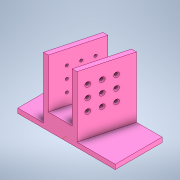
# Autodesk Inventor part: pvcBracketUpperPortion
Saved by Autodesk Inventor 2022.2 (Build 262287000, 287)
## iProperties
Created: 2021-10-20
Part Number: pvcBracketUpperPortion
Material: PC/ABS Plastic
Document SubType Name: Modeling
Designer: robst
Density: 0.357273 g/cm^3
Appearance: Pink
Author: robst
Autodesk Inventor part; units mm, degrees
ref_plane "YZ Plane" through (0, 0, 0) normal (1, 0, 0) x (0, 1, 0)
ref_plane "XZ Plane" through (0, 0, 0) normal (0, 1, 0) x (-1, 0, 0)
ref_plane "XY Plane" through (0, 0, 0) normal (0, 0, 1) x (1, 0, 0)
sketch "Sketch8" plane through (0, 0, 0) normal (0, 1, 0) x (-1, 0, 0)
  line L0 (83, 40) -> (-83, 40)
  line L1 (-83, 40) -> (-83, -40)
  line L2 (-83, -40) -> (83, -40)
  line L3 (83, -40) -> (83, 40)
  line L4 (83, 40) -> (-83, -40) construction
  line L5 (-83, 40) -> (83, -40) construction
  point P0 (0, 0)
  dimension "d28" = 80
  dimension "d29" = 166
  constraints: 12 end point, 2 midpoint, 2 parallel, 1 horizontal, 1 perpendicular
  measures "d28" distance of L2.end L0.start
  measures "d29" distance between parallel lines of L1 L3
extrude "Extrusion8" add sketch "Sketch8" against normal blind 8
sketch "Sketch11" plane through (0, 0, 0) normal (0, 1, 0) x (1, 0, 0)
  line L0 (83, 40) -> (-83, 40) projected
  line L1 (-83, -40) -> (83, -40) projected
  line L2 (-83, 40) -> (-83, -40) projected
  line L3 (83, -40) -> (83, 40) projected
  line L4 (-31.038, -40) -> (-9.602, 40)
  line L5 (-9.602, 40) -> (-17.8842, 40)
  line L6 (-75, 40) -> (75, 40) projected
  line L7 (-17.8842, 40) -> (-39.3202, -40)
  line L8 (-39.3202, -40) -> (-31.038, -40)
  line L9 (-31.038, -40) -> (-31.038, 40) construction
  line L10 (0, -40) -> (0, 40) construction
  line L11 (9.602, -40) -> (31.038, 40)
  line L12 (31.038, 40) -> (39.3202, 40)
  line L13 (39.3202, 40) -> (17.8842, -40)
  line L14 (17.8842, -40) -> (9.602, -40)
  point P0 (0, 0)
  point P1 (0, -40)
  point P2 (0, -40)
  point P3 (-20.32, 0)
  point P4 (0, 0)
  point P5 (20.32, 0)
  point P6 (39.3202, 40)
  point P7 (31.038, 40)
  point P8 (-17.8842, 40)
  dimension "d39" = -15
  dimension "d40" = 8
  dimension "d42" = 8
  dimension "d44" = 20.32
  dimension "d45" = 20.32
  constraints: 20 end point, 5 point on line, 4 midpoint, 3 parallel, 2 horizontal, 1 perpendicular, 8 other
  measures "d39" angle of L4 L9
  measures "d40" distance between parallel lines of L7 L4
  measures "d42" distance between parallel lines of L13 L11
  measures "d44" distance of point (-20.32, 0) point (0, 0)
  measures "d45" distance of point (20.32, 0) point (0, 0)
extrude "Extrusion11" add sketch "Sketch11" along normal blind 104.1375 contours L13 L1 L11 L0 | L4 L1 L7 L0
sketch "Sketch12" plane through (0, 0, 0) normal (0, 1, 0) x (1, 0, 0)
  line L0 (31.038, 40) -> (-9.602, 40) projected
  line L1 (31.038, 40) -> (9.602, -40) projected
  line L2 (-31.038, -40) -> (9.602, -40) projected
  line L3 (-31.038, -40) -> (-9.602, 40) projected
  line L4 (-9.602, 40) -> (31.038, 40)
  line L5 (31.038, 40) -> (9.602, -40)
  line L6 (9.602, -40) -> (-31.038, -40)
  line L7 (-9.602, 40) -> (-31.038, -40) projected
  line L8 (-31.038, -40) -> (-9.602, 40)
  point P0 (0, 0)
  constraints: 8 end point, 3 equal length
extrude "Extrusion12" add sketch "Sketch12" along normal blind 20
sketch "Sketch15" plane through (-39.3202, 0, 40) normal (-0.9659258, 0, -0.258819) x (-0.258819, 0, 0.9659258)
  line L0 (-82.8221, 104.1375) -> (0, 104.1375) projected
  line L1 (0, 0) -> (0, 104.1375) projected
  line L2 (-82.8221, 0) -> (-82.8221, 104.1375) projected
  line L3 (-2.1436, 20) -> (-84.9657, 20) projected
  line L4 (-82.8221, 40) -> (0, 40) construction
  line L5 (-67.8221, 40) -> (-67.8221, 104.1375) construction
  point P0 (-48.8138, 0)
  point P1 (-82.8221, 52.0688)
  point P2 (-47.8221, 40)
  point P3 (-27.8221, 40)
  point P4 (-67.8221, 60)
  point P5 (-47.8221, 60)
  point P6 (-27.8221, 60)
  point P7 (-67.8221, 80)
  point P8 (-47.8221, 80)
  point P9 (-27.8221, 80)
  dimension "d64" = 15
  dimension "d74" = 20
  dimension "d77" = 20
  dimension "d90" = 20
  constraints: 4 end point, 4 point on line, 2 perpendicular, 1 coincident, 1 horizontal, 1 midpoint, 1 vertical, 8 other
  measures "d64" distance from line of point (-82.822, 52.069) L5
  measures "d74" distance of point (-67.822, 40) point (-47.822, 40)
  measures "d77" distance of point (-67.822, 40) point (-67.822, 60)
  measures "d90" distance between parallel lines of L4 L3
hole "HoleForLeftSideOf2x4" at (-21.7665, 40, -25.5111) at (-26.9429, 40, -6.1926) at (-32.1193, 40, 13.1259) at (-26.9429, 60, -6.1926) at (-21.7665, 60, -25.5111) at (-32.1193, 60, 13.1259) at (-32.1193, 80, 13.1259) at (-26.9429, 80, -6.1926) at (-21.7665, 80, -25.5111) direction (0.9659258, 0, 0.258819) diameter 4.496 depth 8 countersink diameter 8.433 countersink angle 82 clearance for "Flat Head Machine Screw (82)" size "#8" standard "Ansi Unified Screw Threads"
sketch "Sketch16" plane through (39.3202, 0, -40) normal (0.9659258, 0, 0.258819) x (0.258819, 0, -0.9659258)
  line L0 (-82.8221, 104.1375) -> (0, 104.1375) projected
  line L1 (0, 0) -> (0, 104.1375) projected
  line L2 (-82.8221, 0) -> (-82.8221, 104.1375) projected
  line L3 (-82.8221, 0) -> (-65.9689, 0) projected
  line L4 (-2.1436, 20) -> (-84.9657, 20) projected
  line L5 (-82.8221, 40) -> (0, 40) construction
  line L6 (-67.8221, 40) -> (-67.8221, 104.1375) construction
  point P0 (-48.8138, 0)
  point P1 (-47.8221, 40)
  point P2 (-27.8221, 40)
  point P3 (-67.8221, 60)
  point P4 (-47.8221, 60)
  point P5 (-27.8221, 60)
  point P6 (-67.8221, 80)
  point P7 (-47.8221, 80)
  point P8 (-27.8221, 80)
  dimension "d80" = 20
  dimension "d81" = 15
  dimension "d84" = 20
  dimension "d87" = 20
  constraints: 4 end point, 4 point on line, 2 perpendicular, 1 coincident, 1 horizontal, 1 vertical, 8 other
  measures "d80" distance between parallel lines of L5 L4
  measures "d81" distance between parallel lines of L6 L2
  measures "d84" distance of point (-67.822, 40) point (-47.822, 40)
  measures "d87" distance of point (-67.822, 40) point (-67.822, 60)
hole "HolesForRightSideOf2x4" at (26.9429, 40, 6.1926) at (32.1193, 40, -13.1259) at (21.7665, 60, 25.5111) at (26.9429, 60, 6.1926) at (32.1193, 60, -13.1259) at (21.7665, 80, 25.5111) at (26.9429, 80, 6.1926) at (32.1193, 80, -13.1259) at (21.7665, 40, 25.5111) direction (-0.9659258, 0, -0.258819) diameter 4.496 depth 8 countersink diameter 8.433 countersink angle 82 clearance for "Flat Head Machine Screw (82)" size "#8" standard "Ansi Unified Screw Threads"
equation "\"d28\" = widthOfBracket"
equation "\"d30\" = wallThickness"
equation "\"d39\" = azimuth"
equation "\"d40\" = wallThickness"
equation "\"d42\" = wallThickness"
equation "\"d44\" = 0.5 * twoByFourWidth"
equation "\"d45\" = 0.5 * twoByFourWidth"
equation "\"d46\" = twoByFourDepth + baseBelowTwoByFour"
equation "\"d49\" = baseBelowTwoByFour"
equation "\"wallThickness\" = 8"
equation "\"widthOfBracket\" = 80"
equation "\"twoByFourWidth\" = 40.64"
equation "\"twoByFourDepth\" = 84.1375"
equation "\"azimuth\" = -15deg"
equation "\"elevation\" = 20deg"
equation "\"baseBelowTwoByFour\" = 20"
equation "\"centerForTwoHoles\" = 0.25 * diagonalLine"
equation "\"depthOfExtrusionForMatingToLowerHalf\" = 12.5"
equation "\"depthForWasherForMatingToCase\" = 14"
equation "\"diagonalLine\" = 85.134222"
body "Solid2"
